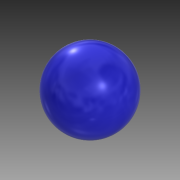
# Autodesk Inventor part: 2022 Cargo
Saved by Autodesk Inventor 2022 (Build 260153000, 153)
## iProperties
Created: 2022-01-10
Part Number: 2022 Cargo
Material: Rubber
Document SubType Name: Modeling
Designer: Desktop
Appearance: Smooth - Red
Surface Area: 1829.29 cm^2
Volume: 7356.95 cm^3
Author: Desktop
Autodesk Inventor part; units mm, degrees
ref_plane "YZ Plane" through (0, 0, 0) normal (1, 0, 0) x (0, 1, 0)
ref_plane "XZ Plane" through (0, 0, 0) normal (0, 1, 0) x (-1, 0, 0)
ref_plane "XY Plane" through (0, 0, 0) normal (0, 0, 1) x (1, 0, 0)
sketch "Sketch1" plane through (0, 0, 0) normal (0, 0, 1) x (1, 0, 0)
  circle A0 centre (0, 0) radius 120.65
  dimension "d0" = 241.3
  constraints: 1 centre point, 1 coincident
  measures "d0" diameter of A0
extrude "Extrusion1" add sketch "Sketch1" along normal mid plane 241.3
fillet "Fillet1" radius 120.65 2 edges at (-120.65, 0, 120.65) (-120.65, 0, -120.65)
thicken "Thicken1" operation add thickness 0.0025 both sides no extend neighbours yes toward (-0.5, -0.8660254, 0) faces at (-60.325, -104.486, 0.0001) (-60.2761, -104.4012, 4.8582) (-60.325, -104.486, -0.0001) (0, 0, 120.65)
body "Solid1"
